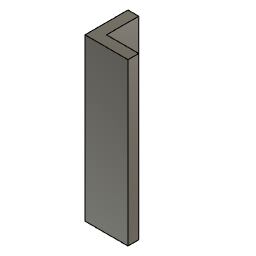
L_Beam v4 (Autodesk Fusion 360 design; units mm, degrees)
Autodesk Fusion 360 part; units mm, degrees
sketch "Sketch1" plane through (0, 0, 0) normal (0, 0, 1) x (1, 0, 0)
  line L0 (0, 0) -> (0, 40)
  line L1 (0, 40) -> (10, 40)
  line L2 (10, 40) -> (10, 10)
  line L3 (10, 10) -> (40, 10)
  line L4 (40, 10) -> (40, 0)
  line L5 (40, 0) -> (0, 0)
  dimension "d1" = 10
  dimension "d2" = 10
  dimension "d3" = 30
  dimension "d4" = 30
  constraint coincident L0.start L5.end
  constraint vertical L0
  constraint perpendicular L0 L1
  constraint perpendicular L1 L2
  constraint perpendicular L0 L3
  constraint perpendicular L3 L4
  constraint perpendicular L0 L5
  measures "d1" distance of L0.end L1.end
  measures "d2" distance of L3.end L4.end
  measures "d3" distance of L1.end L2.end
  measures "d4" distance of L2.end L3.end
extrude "Extrude1" add sketch "Sketch1" along normal blind 150
